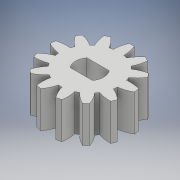
# Autodesk Inventor part: Gear13
Saved by Autodesk Inventor 2018.3 (Build 223284000, 284)
## iProperties
Created: 2019-04-14
Part Number: Gear13
Material: 一般
Document SubType Name: Modeling
Designer: shun2
Density: 1 g/cm^3
Appearance: 既定
Author: shun2
Autodesk Inventor part; units mm, degrees
ref_plane "YZ Plane" through (0, 0, 0) normal (1, 0, 0) x (0, 1, 0)
ref_plane "XZ Plane" through (0, 0, 0) normal (0, 1, 0) x (-1, 0, 0)
ref_plane "XY Plane" through (0, 0, 0) normal (0, 0, 1) x (1, 0, 0)
sketch "スケッチ1" plane through (0, 0, 0) normal (0, 0, 1) x (1, 0, 0)
  arc A0 (-3.88, 6.4184) -> (-3.2378, 4.1327) centre (2.5862, 7.0023) ccw
  arc A1 (-3.2378, 4.1327) -> (-3.7123, 3.7123) centre (0, 0) ccw
  arc A2 (-3.7123, 3.7123) -> (-5.9039, 4.6254) centre (-7.263, -1.7233) ccw
  arc A3 (-5.9039, 4.6254) -> (-6.4184, 3.88) centre (0, 0) ccw
  arc A4 (-6.4184, 3.88) -> (-4.7875, 2.1547) centre (-0.9641, 7.4021) ccw
  arc A5 (-4.7875, 2.1547) -> (-5.0123, 1.5619) centre (0, 0) ccw
  arc A6 (-5.0123, 1.5619) -> (-7.3771, 1.3519) centre (-5.6302, -4.9012) ccw
  arc A7 (-7.3771, 1.3519) -> (-7.4863, 0.4528) centre (0, 0) ccw
  arc A8 (-7.4863, 0.4528) -> (-5.2404, -0.317) centre (-4.2936, 6.1062) ccw
  arc A9 (-5.2404, -0.317) -> (-5.164, -0.9463) centre (0, 0) ccw
  arc A10 (-5.164, -0.9463) -> (-7.1604, -2.2313) centre (-2.7076, -6.9563) ccw
  arc A11 (-7.1604, -2.2313) -> (-6.8392, -3.0781) centre (0, 0) ccw
  arc A12 (-6.8392, -3.0781) -> (-4.4929, -2.716) centre (-6.6395, 3.4114) ccw
  arc A13 (-4.4929, -2.716) -> (-4.1327, -3.2378) centre (0, 0) ccw
  arc A14 (-4.1327, -3.2378) -> (-5.3033, -5.3033) centre (0.8353, -7.4178) ccw
  arc A15 (-5.3033, -5.3033) -> (-4.6254, -5.9039) centre (0, 0) ccw
  arc A16 (-4.6254, -5.9039) -> (-2.716, -4.4929) centre (-7.4644, -0.0649) ccw
  arc A17 (-2.716, -4.4929) -> (-2.1547, -4.7875) centre (0, 0) ccw
  arc A18 (-2.1547, -4.7875) -> (-2.2313, -7.1604) centre (4.1868, -6.1799) ccw
  arc A19 (-2.2313, -7.1604) -> (-1.3519, -7.3771) centre (0, 0) ccw
  arc A20 (-1.3519, -7.3771) -> (-0.317, -5.2404) centre (-6.5792, -3.5263) ccw
  arc A21 (-0.317, -5.2404) -> (0.317, -5.2404) centre (0, 0) ccw
  arc A22 (0.317, -5.2404) -> (1.3519, -7.3771) centre (6.5792, -3.5263) ccw
  arc A23 (1.3519, -7.3771) -> (2.2313, -7.1604) centre (0, 0) ccw
  arc A24 (2.2313, -7.1604) -> (2.1547, -4.7875) centre (-4.1868, -6.1799) ccw
  arc A25 (2.1547, -4.7875) -> (2.716, -4.4929) centre (0, 0) ccw
  arc A26 (2.716, -4.4929) -> (4.6254, -5.9039) centre (7.4644, -0.0649) ccw
  arc A27 (4.6254, -5.9039) -> (5.3033, -5.3033) centre (0, 0) ccw
  arc A28 (5.3033, -5.3033) -> (4.1327, -3.2378) centre (-0.8353, -7.4178) ccw
  arc A29 (4.1327, -3.2378) -> (4.4929, -2.716) centre (0, 0) ccw
  arc A30 (4.4929, -2.716) -> (6.8392, -3.0781) centre (6.6395, 3.4114) ccw
  arc A31 (6.8392, -3.0781) -> (7.1604, -2.2313) centre (0, 0) ccw
  arc A32 (7.1604, -2.2313) -> (5.164, -0.9463) centre (2.7076, -6.9563) ccw
  arc A33 (5.164, -0.9463) -> (5.2404, -0.317) centre (0, 0) ccw
  arc A34 (5.2404, -0.317) -> (7.4863, 0.4528) centre (4.2936, 6.1062) ccw
  arc A35 (7.4863, 0.4528) -> (7.3771, 1.3519) centre (0, 0) ccw
  arc A36 (7.3771, 1.3519) -> (5.0123, 1.5619) centre (5.6302, -4.9012) ccw
  arc A37 (5.0123, 1.5619) -> (4.7875, 2.1547) centre (0, 0) ccw
  arc A38 (4.7875, 2.1547) -> (6.4184, 3.88) centre (0.9641, 7.4021) ccw
  arc A39 (6.4184, 3.88) -> (5.9039, 4.6254) centre (0, 0) ccw
  arc A40 (5.9039, 4.6254) -> (3.7123, 3.7123) centre (7.263, -1.7233) ccw
  arc A41 (3.7123, 3.7123) -> (3.2378, 4.1327) centre (0, 0) ccw
  arc A42 (3.2378, 4.1327) -> (3.88, 6.4184) centre (-2.5862, 7.0023) ccw
  arc A43 (3.88, 6.4184) -> (3.0781, 6.8392) centre (0, 0) ccw
  arc A44 (3.0781, 6.8392) -> (1.5619, 5.0123) centre (7.2319, 1.8493) ccw
  arc A45 (1.5619, 5.0123) -> (0.9463, 5.164) centre (0, 0) ccw
  arc A46 (0.9463, 5.164) -> (0.4528, 7.4863) centre (-5.5441, 4.9983) ccw
  arc A47 (0.4528, 7.4863) -> (-0.4528, 7.4863) centre (0, 0) ccw
  arc A48 (-0.4528, 7.4863) -> (-0.9463, 5.164) centre (5.5441, 4.9983) ccw
  arc A49 (-0.9463, 5.164) -> (-1.5619, 5.0123) centre (0, 0) ccw
  arc A50 (-1.5619, 5.0123) -> (-3.0781, 6.8392) centre (-7.2319, 1.8493) ccw
  arc A51 (-3.0781, 6.8392) -> (-3.88, 6.4184) centre (0, 0) ccw
  constraints: 104 point on circle, 52 centre point
sketch "スケッチ2" plane through (0, 0, 0) normal (0, 0, 1) x (1, 0, 0)
  line L0 (-2, 1.5) -> (2, 1.5)
  line L1 (2, -1.5) -> (-2, -1.5)
  arc A0 (-2, 1.5) -> (-2, -1.5) centre (0, 0) ccw
  arc A1 (2, -1.5) -> (2, 1.5) centre (0, 0) ccw
  point P0 (0, 0)
  point P1 (0, 0)
  point P2 (0, 0)
  point P3 (0, 0)
  point P4 (0, 0)
  point P5 (0, 0)
  point P6 (0, 0)
  point P7 (0, 0)
  point P8 (0, 0)
  point P9 (0, 0)
  point P10 (0, 0)
  point P11 (0, 0)
  point P12 (0, 0)
  point P13 (0, 0)
  point P14 (0, 0)
  point P15 (0, 0)
  point P16 (0, 0)
  point P17 (0, 0)
  point P18 (0, 0)
  point P19 (0, 0)
  point P20 (0, 0)
  point P21 (0, 0)
  point P22 (0, 0)
  point P23 (0, 0)
  point P24 (0, 0)
  point P25 (0, 0)
  constraints: 4 end point, 4 point on circle, 2 centre point, 1 coincident, 1 horizontal, 1 parallel
extrude "押し出し1" add sketch "スケッチ1" along normal blind 6.5
extrude "押し出し2" cut sketch "スケッチ2" along normal blind 6.5
